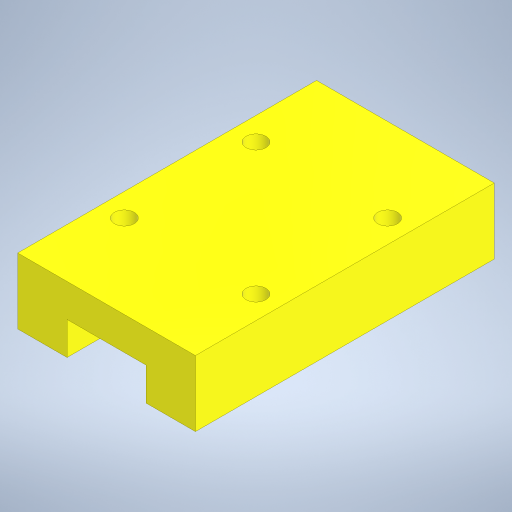
# Autodesk Inventor part: MGN12H_block
Saved by Autodesk Inventor 2024 (Build 280153000, 153)
## iProperties
Created: 2023-08-27
Part Number: MGN12H_block
Material: ABS Plastic
Document SubType Name: Modeling
Designer: l1534
Density: 1.06 g/cm^3
Appearance: Smooth - Yellow
Author: l1534
Autodesk Inventor part; units mm, degrees
ref_plane "YZ Plane" through (0, 0, 0) normal (1, 0, 0) x (0, 1, 0)
ref_plane "XZ Plane" through (0, 0, 0) normal (0, 1, 0) x (-1, 0, 0)
ref_plane "XY Plane" through (0, 0, 0) normal (0, 0, 1) x (1, 0, 0)
sketch "Sketch1" plane through (0, 0, 0) normal (0, 0, 1) x (1, 0, 0)
  line L0 (-8.8498, -2.5153) -> (-8.8498, 7.4847)
  line L1 (-8.8498, 7.4847) -> (18.1502, 7.4847)
  line L2 (18.1502, 7.4847) -> (18.1502, -2.5153)
  line L3 (18.1502, -2.5153) -> (10.6502, -2.5153)
  line L4 (10.6502, -2.5153) -> (10.6502, 2.4847)
  line L5 (10.6502, 2.4847) -> (-1.3498, 2.4847)
  line L6 (-1.3498, 2.4847) -> (-1.3498, -2.5153)
  line L7 (-8.8498, -2.5153) -> (-1.3498, -2.5153)
  point P0 (0, 0)
  dimension "d0" = 12
  dimension "d1" = 27
  dimension "d2" = 7.5
  dimension "d3" = 10
  dimension "d4" = 5
  constraints: 16 end point, 6 perpendicular, 1 horizontal, 1 point on line, 1 vertical
  measures "d0" distance of L4.end L5.end
  measures "d1" distance of L0.end L1.end
  measures "d2" distance of L2.end L3.end
  measures "d3" distance of L1.end L2.end
  measures "d4" distance of L3.end L4.end
extrude "Extrusion1" add sketch "Sketch1" along normal blind 45.4
sketch "Sketch2" plane through (-8.8498, 7.4847, 0) normal (0, 1, 0) x (1, 0, 0)
  circle A0 centre (3.5, -32.7) radius 1.5
  circle A1 centre (23.5, -32.7) radius 1.5
  circle A2 centre (23.5, -12.7) radius 1.5
  circle A3 centre (3.5, -12.7) radius 1.5
  line L0 (0, 0) -> (0, -45.4) projected
  line L1 (27, 0) -> (0, 0) projected
  line L2 (27, -45.4) -> (0, -45.4) projected
  point P0 (8.8498, 0)
  dimension "d7" = 3
  dimension "d8" = 3
  dimension "d9" = 3
  dimension "d10" = 3
  dimension "d11" = 20
  dimension "d12" = 20
  dimension "d13" = 20
  dimension "d14" = 3.5
  dimension "d15" = 12.7
  dimension "d16" = 12.7
  dimension "d17" = 12.7
  dimension "d18" = 12.7
  constraints: 4 centre point
  measures "d7" diameter of A0
  measures "d8" diameter of A1
  measures "d9" diameter of A3
  measures "d10" diameter of A2
  measures "d11" distance of A0.centre A1.centre
  measures "d12" distance of A3.centre A2.centre
  measures "d13" distance of A0.centre A3.centre
  measures "d14" distance from line of L0 A3.centre
  measures "d15" distance from line of L1 A3.centre
  measures "d16" distance from line of L1 A2.centre
  measures "d17" distance from line of L2 A0.centre
  measures "d18" distance from line of L2 A1.centre
extrude "Extrusion2" cut sketch "Sketch2" against normal through all
body "Solid1"
